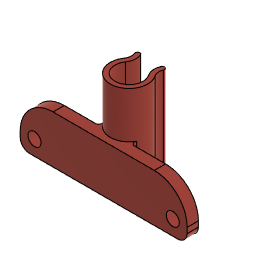
openMV Mount v2 (Autodesk Fusion 360 design; units mm, degrees)
Autodesk Fusion 360 part; units mm, degrees
note: some values were not read from the file. Chosen so that the rebuilt part matches the saved one: which face or edge a step refers to.
sketch "Sketch1" plane through (0, 0, 0) normal (0, 0, 1) x (1, 0, 0)
  line L0 (17.78, -1.2) -> (-17.78, -1.2)
  line L1 (-17.78, -1.2) -> (-17.78, 1.2)
  line L2 (-17.78, 1.2) -> (17.78, 1.2)
  line L3 (17.78, 1.2) -> (17.78, -1.2)
  line L4 (17.78, -1.2) -> (-17.78, 1.2) construction
  line L5 (-17.78, -1.2) -> (17.78, 1.2) construction
  arc A0 (-2.4575, 5.9207) -> (2.4575, 5.9207) centre (0, 4.2) ccw
  line L6 (0, -1.2) -> (0, 10.932)
  line L7 (0, 4.2) -> (3, 4.2) construction
  line L8 (0, 4.2) -> (2.4575, 5.9207) construction
  arc A1 (2.4575, 9.3622) -> (2.4575, 5.9207) centre (4.9149, 7.6415) ccw
  arc A2 (-2.4575, 5.9207) -> (-2.4575, 9.3622) centre (-4.9149, 7.6415) ccw
  dimension "d1" = 35.56
  dimension "d2" = 2.4
  dimension "d3" = 3
  dimension "d4" = 35
  dimension "d5" = 3
  constraint horizontal L0
  constraint perpendicular L0 L1
  constraint parallel L0 L2
  constraint parallel L1 L3
  constraint coincident L4 origin
  constraint coincident L5 origin
  constraint midpoint L0 L6.start
  constraint perpendicular L0 L6
  constraint tangent L2 A0
  constraint coincident A0.centre L7.start
  constraint coincident A0 L7.end
  constraint horizontal L7
  constraint symmetric A0.start A0.end L6
  constraint vertical A0.end A1.start
  constraint tangent A0 A1
  constraint symmetric A0.end L6 A0.start
  constraint symmetric L6 A1.start A2.end
  constraint symmetric L6 A1 A2
  measures "d1" distance of L1.end L2.end
  measures "d2" distance of L0.end L1.end
  measures "d3" radius of A0
  measures "d4" angle of L7 L8
  measures "d5" radius of A1
extrude "Extrude1" add sketch "Sketch1" along normal blind 10.16
extrude "Extrude2" add sketch "Sketch1" along normal blind 20 thin wall 1 on the left open curves A2 A0 A1
fillet "Fillet1" radius 0.5 2 edges at (-2.4575, 9.3622, 10) (-3.2766, 8.7886, 10)
fillet "Fillet1" radius 0.5 2 edges at (3.2766, 8.7886, 10) (2.4575, 9.3622, 10)
fillet "Fillet2" radius 0.75 2 edges at (2.6458, 1.2, 5.08) (-2.6458, 1.2, 5.08)
sketch "Sketch2" plane through (0, -1.2, 0) normal (0, -1, 0) x (1, 0, 0)
  line L0 (-17.78, 0) -> (17.78, 0)
  line L1 (17.78, 0) -> (17.78, 10.16)
  line L2 (17.78, 10.16) -> (-17.78, 10.16)
  line L3 (-17.78, 10.16) -> (-17.78, 0)
  line L4 (0, 0) -> (0, 10.16)
  circle A0 centre (14.732, 3.175) radius 1.397
  circle A1 centre (-14.732, 3.175) radius 1.397
  line L5 (17.78, 0) -> (-17.78, 0)
  dimension "d13" = 2.794
  dimension "d14" = 2.794
  dimension "d15" = 29.464
  dimension "d16" = 3.175
  constraint coincident L4.start origin
  constraint midpoint L2 L4.end
  constraint symmetric L4 A0 A1
  measures "d13" diameter of A0
  measures "d14" diameter of A1
  measures "d15" distance of A0.centre A1.centre
  measures "d16" distance of A0.centre L5
extrude "Extrude3" cut sketch "Sketch2" against normal blind 2.4 contours A0 | A1
fillet "Fillet3" radius 7 2 edges at (17.78, 0, 10.16) (-17.78, 0, 10.16)
fillet "Fillet4" radius 2 2 edges at (17.78, 0, 0) (-17.78, 0, 0)
equation "d5 = d3"
equation "d6 = 1.75 in - 1.35 in"
equation "d14 = d13"
